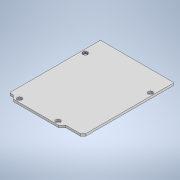
# Autodesk Inventor part: ArduinoUnoFootprintPART
Saved by Autodesk Inventor 2021 (Build 250183000, 183)
## iProperties
Created: 2020-09-24
Part Number: ArduinoUnoFootprintPART
Material: Generic
Document SubType Name: Modeling
Designer: dech3
Density: 1 g/cm^3
Appearance: Default
Author: dech3
Autodesk Inventor part; units mm, degrees
ref_plane "YZ Plane" through (0, 0, 0) normal (1, 0, 0) x (0, 1, 0)
ref_plane "XZ Plane" through (0, 0, 0) normal (0, 1, 0) x (-1, 0, 0)
ref_plane "XY Plane" through (0, 0, 0) normal (0, 0, 1) x (1, 0, 0)
sketch "Sketch1" plane through (0, 0, 0) normal (0, 1, 0) x (-1, 0, 0)
  line L0 (26, -28) -> (-27.5, -28)
  line L1 (-27.5, -28) -> (-27.5, 38.15)
  line L2 (26, 38.15) -> (26, -28)
  line L3 (26, 38.15) -> (23.15, 38.15)
  line L4 (23.15, 38.15) -> (20.59, 40.75)
  line L5 (20.59, 40.75) -> (-12.27, 40.75)
  line L6 (-12.27, 40.75) -> (-14.9, 38.15)
  line L7 (-14.9, 38.15) -> (-27.5, 38.15)
  point P0 (0, 0)
  point P1 (-27.5, 40.75)
  point P2 (26, 40.75)
  point P3 (4.16, 40.75)
  point P4 (24.575, 38.15)
  point P5 (-21.2, 38.15)
  dimension "d2" = 53.5
  dimension "d12" = 68.75
  dimension "d13" = 2.6
  dimension "d14" = 2.85
  dimension "d15" = 2.56
  dimension "d16" = 32.86
  dimension "d17" = 12.6
  dimension "d18" = 28
  dimension "d19" = 26
  constraints: 16 end point, 7 coincident, 5 horizontal alignment, 3 horizontal, 3 midpoint, 2 vertical alignment, 1 parallel, 1 perpendicular
  measures "d2" distance between parallel lines of L2 L1
  measures "d12" distance between parallel lines of L5 L0
  measures "d13" distance from line of point (24.575, 38.15) L5
  measures "d14" distance from line of L3.end L2
  measures "d15" horizontal distance of L4.end L3.end
  measures "d16" distance of L5.end L4.end
  measures "d17" distance of L1.end L6.end
  measures "d18" distance from line of L0 point (0, 0)
  measures "d19" distance from line of L2 point (0, 0)
extrude "Extrusion1" add sketch "Sketch1" along normal blind 1.6
chamfer "Chamfer1" distance 2 angle 45 1 edges at (27.5, 0.8, 38.15)
chamfer "Chamfer2" distance 0.5 angle 45 3 edges at (-26, 0.8, 38.15) (-26, 0.8, -28) (27.5, 0.8, -28)
sketch "Sketch2" plane through (0, 1.6, 0) normal (0, 1, 0) x (1, 0, 0)
  line L0 (-26, 27.5) -> (-26, -37.65) projected
  line L1 (27, 28) -> (-25.5, 28) projected
  line L2 (27.5, -36.15) -> (27.5, 27.5) projected
  line L3 (-20.59, -40.75) -> (12.27, -40.75) projected
  point P0 (0, 0)
  point P1 (-23.3, 14.21)
  point P2 (25.32, 13)
  point P3 (9.5, -38.37)
  point P4 (-18.52, -38.37)
  dimension "d28" = 2.7
  dimension "d29" = 13.79
  dimension "d30" = 2.18
  dimension "d31" = 15
  dimension "d32" = 7.48
  dimension "d33" = 2.38
  dimension "d34" = 18
  constraints: 1 horizontal alignment
  measures "d28" distance from line of L0 point (-23.3, 14.21)
  measures "d29" distance from line of L1 point (-23.3, 14.21)
  measures "d30" distance from line of L2 point (25.32, 13)
  measures "d31" distance from line of L1 point (25.32, 13)
  measures "d32" distance from line of L0 point (-18.52, -38.37)
  measures "d33" distance from line of L3 point (-18.52, -38.37)
  measures "d34" distance from line of L2 point (9.5, -38.37)
hole "Hole1" at (-23.3, 1.6, -14.21) at (25.32, 1.6, -13) at (9.5, 1.6, 38.37) at (-18.52, 1.6, 38.37) direction (0, -1, 0) diameter 3.4 end through all clearance for "Countersunk Flat Head Screw ISO 2009/7046" size "M3" standard "ISO"
body "Solid1"
